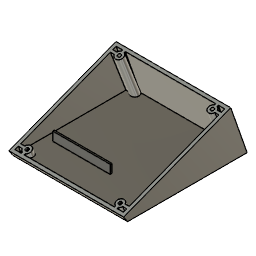
Waveshare_86_21deg_v0.9_CODEX_DRAFT (Autodesk Fusion 360 design; units mm, degrees)
part number: 2026-09-02-16-15-16-232
part number: 2026-09-02-16-15-18-443
part number: 2026-09-02-16-21-17-186
Autodesk Fusion 360 part; units mm, degrees
(part 1 of 4)
sketch "草图1" plane through (0, 0, 0) normal (1, 0, 0) x (0, 0, -1) in component "01_Integrated_Support_PRINT_BODY"
  line L0 (0, 3) -> (0, 93.1088)
  line L1 (0, 93.1088) -> (-35.4988, 80.7547)
  line L2 (-35.4988, 80.7547) -> (-4.5, 0)
  line L3 (-4.5, 0) -> (0, 3)
  line L4 (0, 0) -> (0, 3) construction
  line L5 (0, 0) -> (0, 93.1088) construction
  line L6 (0, 0) -> (-4.5, 0) construction
  dimension "d35" = 3
  dimension "d36" = 93.1088
  dimension "d37" = 35.4988
  dimension "d38" = 80.7547
  dimension "d39" = 4.5
  constraint vertical L4
  constraint vertical L5
  constraint horizontal L6
  measures "d35" vertical distance of L4.start L0.start
  measures "d36" vertical distance of L4.start L0.end
  measures "d37" horizontal distance of L4.start L1.end
  measures "d38" vertical distance of L4.start L1.end
  measures "d39" horizontal distance of L4.start L2.end
extrude "02_Outer_Envelope" add sketch "草图1" along normal blind 86.5 makes body 1 in component "01_Integrated_Support_PRINT_BODY"
extrude "03_Envelope_Reference_Tool" add sketch "草图1" along normal blind 86.5 separate body makes body 2 in component "01_Integrated_Support_PRINT_BODY"
shell "04_Open_Top_Integrated_Floor_No_Flange" thickness 2.4 removed faces 1 at (57.6667, 53.8365, 25.1659) on bodies 1 in component "01_Integrated_Support_PRINT_BODY"
ref_plane "工作平面1" through (12.125, 0, 0) normal (0, -0.358368, 0.93358) x (1, 0, 0) in component "01_Integrated_Support_PRINT_BODY"
ref_plane "工作平面2" through (12.125, -1.5055, 3.9221) normal (0, -0.358368, 0.93358) x (1, 0, 0) in component "01_Integrated_Support_PRINT_BODY"
sketch "草图2" plane through (0, -1.5055, 3.9221) normal (0, -0.358368, 0.93358) x (1, 0, 0) in component "01_Integrated_Support_PRINT_BODY"
  circle A0 centre (8.2, 7.7127) radius 3
  dimension "d49" = 8.2
  dimension "d50" = 7.7127
  dimension "d51" = 6
  measures "d49" horizontal distance of origin A0.centre
  measures "d50" vertical distance of origin A0.centre
  measures "d51" diameter of A0
extrude "BossSolid_FrontL" add sketch "草图2" against normal blind 70 separate body makes body 3 in component "01_Integrated_Support_PRINT_BODY"
sketch "草图4" plane through (0, -1.5055, 3.9221) normal (0, -0.358368, 0.93358) x (1, 0, 0) in component "01_Integrated_Support_PRINT_BODY"
  line L0 (0, 6.7127) -> (8.2, 6.7127)
  line L1 (8.2, 6.7127) -> (8.2, 8.7127)
  line L2 (8.2, 8.7127) -> (0, 8.7127)
  line L3 (0, 8.7127) -> (0, 6.7127)
  line L4 (0, 0) -> (0, 6.7127) construction
  dimension "d56" = 6.7127
  dimension "d57" = 8.2
  dimension "d58" = 2
  constraint horizontal L0
  constraint horizontal L2
  constraint vertical L1
  constraint vertical L3
  constraint vertical L4
  measures "d56" vertical distance of L4.start L0.start
  measures "d57" horizontal distance of L0.start L0.end
  measures "d58" vertical distance of L0.end L1.end
extrude "WebSolid_FrontL" add sketch "草图4" against normal blind 70 separate body makes body 4 in component "01_Integrated_Support_PRINT_BODY"
sketch "草图5" plane through (0, -1.5055, 3.9221) normal (0, -0.358368, 0.93358) x (1, 0, 0) in component "01_Integrated_Support_PRINT_BODY"
  circle A0 centre (78.3, 7.7127) radius 3
  dimension "d61" = 78.3
  dimension "d62" = 7.7127
  dimension "d63" = 6
  measures "d61" horizontal distance of origin A0.centre
  measures "d62" vertical distance of origin A0.centre
  measures "d63" diameter of A0
extrude "BossSolid_FrontR" add sketch "草图5" against normal blind 70 separate body makes body 5 in component "01_Integrated_Support_PRINT_BODY"
sketch "草图6" plane through (0, -1.5055, 3.9221) normal (0, -0.358368, 0.93358) x (1, 0, 0) in component "01_Integrated_Support_PRINT_BODY"
  line L0 (78.3, 6.7127) -> (86.5, 6.7127)
  line L1 (86.5, 6.7127) -> (86.5, 8.7127)
  line L2 (86.5, 8.7127) -> (78.3, 8.7127)
  line L3 (78.3, 8.7127) -> (78.3, 6.7127)
  dimension "d66" = 78.3
  dimension "d67" = 6.7127
  dimension "d68" = 8.2
  dimension "d69" = 2
  constraint horizontal L0
  constraint horizontal L2
  constraint vertical L1
  constraint vertical L3
  measures "d66" horizontal distance of origin L0.start
  measures "d67" vertical distance of origin L0.start
  measures "d68" horizontal distance of L0.start L0.end
  measures "d69" vertical distance of L0.end L1.end
extrude "WebSolid_FrontR" add sketch "草图6" against normal blind 70 separate body makes body 6 in component "01_Integrated_Support_PRINT_BODY"
sketch "草图7" plane through (0, -1.5055, 3.9221) normal (0, -0.358368, 0.93358) x (1, 0, 0) in component "01_Integrated_Support_PRINT_BODY"
  circle A0 centre (8.2, 82.0127) radius 3
  dimension "d72" = 8.2
  dimension "d73" = 82.0127
  dimension "d74" = 6
  measures "d72" horizontal distance of origin A0.centre
  measures "d73" vertical distance of origin A0.centre
  measures "d74" diameter of A0
extrude "BossSolid_RearL" add sketch "草图7" against normal blind 70 separate body makes body 7 in component "01_Integrated_Support_PRINT_BODY"
sketch "草图8" plane through (0, -1.5055, 3.9221) normal (0, -0.358368, 0.93358) x (1, 0, 0) in component "01_Integrated_Support_PRINT_BODY"
  line L0 (0, 81.0127) -> (8.2, 81.0127)
  line L1 (8.2, 81.0127) -> (8.2, 83.0127)
  line L2 (8.2, 83.0127) -> (0, 83.0127)
  line L3 (0, 83.0127) -> (0, 81.0127)
  line L4 (0, 0) -> (0, 81.0127) construction
  dimension "d77" = 81.0127
  dimension "d78" = 8.2
  dimension "d79" = 2
  constraint horizontal L0
  constraint horizontal L2
  constraint vertical L1
  constraint vertical L3
  constraint vertical L4
  measures "d77" vertical distance of L4.start L0.start
  measures "d78" horizontal distance of L0.start L0.end
  measures "d79" vertical distance of L0.end L1.end
extrude "WebSolid_RearL" add sketch "草图8" against normal blind 70 separate body makes body 8 in component "01_Integrated_Support_PRINT_BODY"
sketch "草图9" plane through (0, -1.5055, 3.9221) normal (0, -0.358368, 0.93358) x (1, 0, 0) in component "01_Integrated_Support_PRINT_BODY"
  circle A0 centre (78.3, 82.0127) radius 3
  dimension "d82" = 78.3
  dimension "d83" = 82.0127
  dimension "d84" = 6
  measures "d82" horizontal distance of origin A0.centre
  measures "d83" vertical distance of origin A0.centre
  measures "d84" diameter of A0
extrude "BossSolid_RearR" add sketch "草图9" against normal blind 70 separate body makes body 9 in component "01_Integrated_Support_PRINT_BODY"
sketch "草图10" plane through (0, -1.5055, 3.9221) normal (0, -0.358368, 0.93358) x (1, 0, 0) in component "01_Integrated_Support_PRINT_BODY"
  line L0 (78.3, 81.0127) -> (86.5, 81.0127)
  line L1 (86.5, 81.0127) -> (86.5, 83.0127)
  line L2 (86.5, 83.0127) -> (78.3, 83.0127)
  line L3 (78.3, 83.0127) -> (78.3, 81.0127)
  dimension "d87" = 78.3
  dimension "d88" = 81.0127
  dimension "d89" = 8.2
  dimension "d90" = 2
  constraint horizontal L0
  constraint horizontal L2
  constraint vertical L1
  constraint vertical L3
  measures "d87" horizontal distance of origin L0.start
  measures "d88" vertical distance of origin L0.start
  measures "d89" horizontal distance of L0.start L0.end
  measures "d90" vertical distance of L0.end L1.end
extrude "WebSolid_RearR" add sketch "草图10" against normal blind 70 separate body makes body 10 in component "01_Integrated_Support_PRINT_BODY"
combine "05_Four_Bosses_With_Sidewall_Webs" operation add target body 1 tool bodies 3 4 5 6 7 8 9 10 in component "01_Integrated_Support_PRINT_BODY"
combine "06_Trim_Reinforcement_To_Exact_Envelope" operation intersect target body 1 tool bodies 2 keep tools in component "01_Integrated_Support_PRINT_BODY"
ref_plane "工作平面3" through (12.125, -0.538, 1.4014) normal (0, -0.358368, 0.93358) x (1, 0, 0) in component "01_Integrated_Support_PRINT_BODY"
ref_plane "工作平面4" through (12.125, 8.4212, -21.9381) normal (0, -0.358368, 0.93358) x (1, 0, 0) in component "01_Integrated_Support_PRINT_BODY"
sketch "草图11" plane through (0, -1.5055, 3.9221) normal (0, -0.358368, 0.93358) x (1, 0, 0) in component "01_Integrated_Support_PRINT_BODY"
  circle A0 centre (8.2, 7.7127) radius 1.2
  dimension "d97" = 8.2
  dimension "d98" = 7.7127
  dimension "d99" = 2.4
  measures "d97" horizontal distance of origin A0.centre
  measures "d98" vertical distance of origin A0.centre
  measures "d99" diameter of A0
extrude "07_M2_Through_FrontL" cut sketch "草图11" against normal blind 70 bodies 1 in component "01_Integrated_Support_PRINT_BODY"
sketch "草图12" plane through (0, -0.538, 1.4014) normal (0, -0.358368, 0.93358) x (1, 0, 0) in component "01_Integrated_Support_PRINT_BODY"
  circle A0 centre (8.2, 7.7127) radius 2.2
  dimension "d102" = 8.2
  dimension "d103" = 7.7127
  dimension "d104" = 4.4
  measures "d102" horizontal distance of origin A0.centre
  measures "d103" vertical distance of origin A0.centre
  measures "d104" diameter of A0
extrude "08_Recessed_Socket_Head_FrontL" [suppressed] in component "01_Integrated_Support_PRINT_BODY"
sketch "草图13" plane through (0, -1.5055, 3.9221) normal (0, -0.358368, 0.93358) x (1, 0, 0) in component "01_Integrated_Support_PRINT_BODY"
  circle A0 centre (78.3, 7.7127) radius 1.2
  dimension "d107" = 78.3
  dimension "d108" = 7.7127
  dimension "d109" = 2.4
  measures "d107" horizontal distance of origin A0.centre
  measures "d108" vertical distance of origin A0.centre
  measures "d109" diameter of A0
extrude "07_M2_Through_FrontR" cut sketch "草图13" against normal blind 70 bodies 1 in component "01_Integrated_Support_PRINT_BODY"
sketch "草图14" plane through (0, -0.538, 1.4014) normal (0, -0.358368, 0.93358) x (1, 0, 0) in component "01_Integrated_Support_PRINT_BODY"
  circle A0 centre (78.3, 7.7127) radius 2.2
  dimension "d112" = 78.3
  dimension "d113" = 7.7127
  dimension "d114" = 4.4
  measures "d112" horizontal distance of origin A0.centre
  measures "d113" vertical distance of origin A0.centre
  measures "d114" diameter of A0
extrude "08_Recessed_Socket_Head_FrontR" [suppressed] in component "01_Integrated_Support_PRINT_BODY"
sketch "草图15" plane through (0, -1.5055, 3.9221) normal (0, -0.358368, 0.93358) x (1, 0, 0) in component "01_Integrated_Support_PRINT_BODY"
  circle A0 centre (8.2, 82.0127) radius 1.2
  dimension "d117" = 8.2
  dimension "d118" = 82.0127
  dimension "d119" = 2.4
  measures "d117" horizontal distance of origin A0.centre
  measures "d118" vertical distance of origin A0.centre
  measures "d119" diameter of A0
extrude "07_M2_Through_RearL" cut sketch "草图15" against normal blind 70 bodies 1 in component "01_Integrated_Support_PRINT_BODY"
sketch "草图16" plane through (0, 8.4212, -21.9381) normal (0, -0.358368, 0.93358) x (1, 0, 0) in component "01_Integrated_Support_PRINT_BODY"
  circle A0 centre (8.2, 82.0127) radius 2.2
  dimension "d122" = 8.2
  dimension "d123" = 82.0127
  dimension "d124" = 4.4
  measures "d122" horizontal distance of origin A0.centre
  measures "d123" vertical distance of origin A0.centre
  measures "d124" diameter of A0
extrude "08_Recessed_Socket_Head_RearL" [suppressed] in component "01_Integrated_Support_PRINT_BODY"
sketch "草图17" plane through (0, -1.5055, 3.9221) normal (0, -0.358368, 0.93358) x (1, 0, 0) in component "01_Integrated_Support_PRINT_BODY"
  circle A0 centre (78.3, 82.0127) radius 1.2
  dimension "d127" = 78.3
  dimension "d128" = 82.0127
  dimension "d129" = 2.4
  measures "d127" horizontal distance of origin A0.centre
  measures "d128" vertical distance of origin A0.centre
  measures "d129" diameter of A0
extrude "07_M2_Through_RearR" cut sketch "草图17" against normal blind 70 bodies 1 in component "01_Integrated_Support_PRINT_BODY"
sketch "草图18" plane through (0, 8.4212, -21.9381) normal (0, -0.358368, 0.93358) x (1, 0, 0) in component "01_Integrated_Support_PRINT_BODY"
  circle A0 centre (78.3, 82.0127) radius 2.2
  dimension "d132" = 78.3
  dimension "d133" = 82.0127
  dimension "d134" = 4.4
  measures "d132" horizontal distance of origin A0.centre
  measures "d133" vertical distance of origin A0.centre
  measures "d134" diameter of A0
extrude "08_Recessed_Socket_Head_RearR" [suppressed] in component "01_Integrated_Support_PRINT_BODY"
sketch "草图1 (2)" plane through (0, -1.5055, 3.9221) normal (0, -0.358368, 0.93358) x (1, 0, 0) in component "02_REFERENCE_ORIGINAL_BOX_NOT_FOR_PRINT"
  line L0 (0, 1.6127) -> (86.5, 1.6127)
  line L1 (86.5, 1.6127) -> (86.5, 88.1127)
  line L2 (86.5, 88.1127) -> (0, 88.1127)
  line L3 (0, 88.1127) -> (0, 1.6127)
  line L4 (0, 0) -> (0, 1.6127) construction
  dimension "d137" = 1.6127
  dimension "d138" = 86.5
  dimension "d139" = 86.5
  constraint horizontal L0
  constraint horizontal L2
  constraint vertical L1
  constraint vertical L3
  constraint vertical L4
  measures "d137" vertical distance of L4.start L0.start
  measures "d138" horizontal distance of L0.start L0.end
  measures "d139" vertical distance of L0.end L1.end
extrude "REFERENCE_14mm_Device_Envelope" add sketch "草图1 (2)" along normal blind 14 separate body makes body 11 in component "02_REFERENCE_ORIGINAL_BOX_NOT_FOR_PRINT"
sketch "草图19" plane through (0, -1.5055, 3.9221) normal (0, -0.358368, 0.93358) x (1, 0, 0) in component "01_Integrated_Support_PRINT_BODY"
  line L0 (7.2, 1.6127) -> (9.2, 1.6127)
  line L1 (9.2, 1.6127) -> (9.2, 5.0127)
  line L2 (9.2, 5.0127) -> (7.2, 5.0127)
  line L3 (7.2, 5.0127) -> (7.2, 1.6127)
  dimension "d143" = 7.2
  dimension "d144" = 1.6127
  dimension "d145" = 2
  dimension "d146" = 3.4
  constraint horizontal L0
  constraint horizontal L2
  constraint vertical L1
  constraint vertical L3
  measures "d143" horizontal distance of origin L0.start
  measures "d144" vertical distance of origin L0.start
  measures "d145" horizontal distance of L0.start L0.end
  measures "d146" vertical distance of L0.end L1.end
extrude "EndWall_Reinforcement_FrontL" add sketch "草图19" against normal blind 70 separate body makes body 12 in component "01_Integrated_Support_PRINT_BODY"
sketch "草图20" plane through (0, -1.5055, 3.9221) normal (0, -0.358368, 0.93358) x (1, 0, 0) in component "01_Integrated_Support_PRINT_BODY"
  line L0 (77.3, 1.6127) -> (79.3, 1.6127)
  line L1 (79.3, 1.6127) -> (79.3, 5.0127)
  line L2 (79.3, 5.0127) -> (77.3, 5.0127)
  line L3 (77.3, 5.0127) -> (77.3, 1.6127)
  dimension "d149" = 77.3
  dimension "d150" = 1.6127
  dimension "d151" = 2
  dimension "d152" = 3.4
  constraint horizontal L0
  constraint horizontal L2
  constraint vertical L1
  constraint vertical L3
  measures "d149" horizontal distance of origin L0.start
  measures "d150" vertical distance of origin L0.start
  measures "d151" horizontal distance of L0.start L0.end
  measures "d152" vertical distance of L0.end L1.end
extrude "EndWall_Reinforcement_FrontR" add sketch "草图20" against normal blind 70 separate body makes body 13 in component "01_Integrated_Support_PRINT_BODY"
sketch "草图21" plane through (0, -1.5055, 3.9221) normal (0, -0.358368, 0.93358) x (1, 0, 0) in component "01_Integrated_Support_PRINT_BODY"
  line L0 (7.2, 84.7127) -> (9.2, 84.7127)
  line L1 (9.2, 84.7127) -> (9.2, 88.1127)
  line L2 (9.2, 88.1127) -> (7.2, 88.1127)
  line L3 (7.2, 88.1127) -> (7.2, 84.7127)
  dimension "d155" = 7.2
  dimension "d156" = 84.7127
  dimension "d157" = 2
  dimension "d158" = 3.4
  constraint horizontal L0
  constraint horizontal L2
  constraint vertical L1
  constraint vertical L3
  measures "d155" horizontal distance of origin L0.start
  measures "d156" vertical distance of origin L0.start
  measures "d157" horizontal distance of L0.start L0.end
  measures "d158" vertical distance of L0.end L1.end
extrude "EndWall_Reinforcement_RearL" add sketch "草图21" against normal blind 70 separate body makes body 14 in component "01_Integrated_Support_PRINT_BODY"
sketch "草图22" plane through (0, -1.5055, 3.9221) normal (0, -0.358368, 0.93358) x (1, 0, 0) in component "01_Integrated_Support_PRINT_BODY"
  line L0 (77.3, 84.7127) -> (79.3, 84.7127)
  line L1 (79.3, 84.7127) -> (79.3, 88.1127)
  line L2 (79.3, 88.1127) -> (77.3, 88.1127)
  line L3 (77.3, 88.1127) -> (77.3, 84.7127)
  dimension "d161" = 77.3
  dimension "d162" = 84.7127
  dimension "d163" = 2
  dimension "d164" = 3.4
  constraint horizontal L0
  constraint horizontal L2
  constraint vertical L1
  constraint vertical L3
  measures "d161" horizontal distance of origin L0.start
  measures "d162" vertical distance of origin L0.start
  measures "d163" horizontal distance of L0.start L0.end
  measures "d164" vertical distance of L0.end L1.end
extrude "EndWall_Reinforcement_RearR" add sketch "草图22" against normal blind 70 separate body makes body 15 in component "01_Integrated_Support_PRINT_BODY"
combine "09_End_Wall_Braces_No_Hole_Overlap" operation add target body 1 tool bodies 12 13 14 15 in component "01_Integrated_Support_PRINT_BODY"
combine "10_Final_Envelope_Trim" operation intersect target body 1 tool bodies 2 keep tools in component "01_Integrated_Support_PRINT_BODY"
sketch "草图24" plane through (0, 0, 0) normal (0, 0, 1) x (1, 0, 0) in component "01_Integrated_Support_PRINT_BODY"